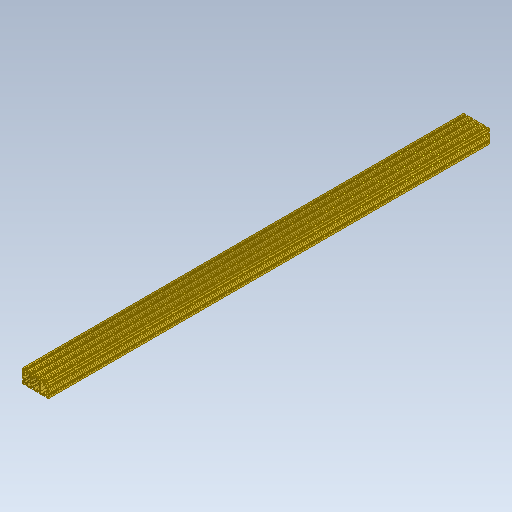
# Autodesk Inventor part: Perfil 60×120 12 rasgos_AST06012012
Saved by Autodesk Inventor 2025.2 (Build 292293000, 293)
## iProperties
Created: 2025-04-07
Part Number: Perfil 60×120 12 rasgos_AST06012012
Material: Ouro
Document SubType Name: Modeling
Designer: Gustavo Sousa
Density: 19.3 g/cm^3
Appearance: Metal quente 2400F
Author: Gustavo Sousa
Autodesk Inventor part; units mm, degrees
ref_plane "YZ Plane" through (0, 0, 0) normal (1, 0, 0) x (0, 1, 0)
ref_plane "XZ Plane" through (0, 0, 0) normal (0, 1, 0) x (-1, 0, 0)
ref_plane "XY Plane" through (0, 0, 0) normal (0, 0, 1) x (1, 0, 0)
sketch "Esboço1" plane through (0, 0, 0) normal (0, 0, 1) x (1, 0, 0)
  line L0 (-60, 30) -> (60, 30) construction
  line L1 (-60, 30) -> (-60, -30) construction
  line L2 (-60, 30) -> (0, 30) construction
  line L3 (-60, 30) -> (-60, 0) construction
  circle A0 centre (-45, 15) radius 5
  line L4 (-45, 15) -> (-60, 30) construction
  line L5 (-60, 30) -> (-30, 30) construction
  line L6 (-52, 22) -> (-38, 22) construction
  line L7 (-49.1, 30) -> (-40.9, 30) construction
  line L8 (-45, 15) -> (-30, 30) construction
  line L9 (-38, 22) -> (-38, 15) construction
  line L10 (-49.1, 30) -> (-49.6, 30) construction
  line L11 (-49.6, 30) -> (-49.6, 29.5)
  line L12 (-49.6, 29.5) -> (-49.1, 29.5)
  line L13 (-49.1, 29.5) -> (-49.1, 30) construction
  line L14 (-49.1, 30) -> (-49.1, 27.8) construction
  line L15 (-49.1, 27.8) -> (-56.2444, 27.8) construction
  arc A1 (-59.5, 30) -> (-60, 29.5) centre (-59.5, 29.5) ccw
  line L16 (-56.2444, 27.8) -> (-50.4444, 22) construction
  arc A2 (-55.0373, 27.8) -> (-55.3908, 26.9464) centre (-55.0373, 27.3) ccw
  arc A3 (-50.5908, 22.1464) -> (-50.2373, 22) centre (-50.2373, 22.5) ccw
  line L17 (-55.0373, 27.8) -> (-49.1, 27.8)
  line L18 (-55.3908, 26.9464) -> (-50.5908, 22.1464)
  line L19 (-50.2373, 22) -> (-45, 22)
  line L20 (-59.5, 30) -> (-49.6, 30)
  line L21 (-39.5556, 22) -> (-33.7556, 27.8) construction
  line L22 (-40.9, 30) -> (-40.4, 30) construction
  line L23 (-40.4, 30) -> (-40.4, 29.5)
  line L24 (-40.4, 29.5) -> (-40.9, 29.5)
  line L25 (-40.9, 29.5) -> (-40.9, 30) construction
  line L26 (-40.9, 30) -> (-40.9, 27.8) construction
  line L27 (-40.9, 27.8) -> (-33.7556, 27.8) construction
  arc A4 (-34.6092, 26.9464) -> (-34.9627, 27.8) centre (-34.9627, 27.3) ccw
  line L28 (-49.1, 29.5) -> (-49.1, 27.8)
  line L29 (-40.9, 29.5) -> (-40.9, 27.8)
  arc A5 (-39.7627, 22) -> (-39.4092, 22.1464) centre (-39.7627, 22.5) ccw
  line L30 (-45, 22) -> (-39.7627, 22)
  line L31 (-39.4092, 22.1464) -> (-34.6092, 26.9464)
  line L32 (-34.9627, 27.8) -> (-40.9, 27.8)
  line L33 (-30, 30) -> (-30, 28.4444) construction
  line L34 (-38, 15) -> (-40, 15) construction
  line L35 (-38, 20.4444) -> (-30, 28.4444) construction
  line L36 (-38, 20.4444) -> (-38, 15) construction
  line L37 (-45, 20) -> (-45, 22)
  line L38 (-40.4, 30) -> (-30, 30)
  arc A6 (-37.8536, 20.5908) -> (-38, 20.2373) centre (-37.5, 20.2373) ccw
  line L39 (-38, 20.2373) -> (-38, 15)
  line L40 (-37.8536, 20.5908) -> (-30, 28.4444)
  arc A7 (-40, 15) -> (-38, 15) centre (-39, 15) ccw
  line L41 (-52, 22) -> (-52, 15) construction
  line L42 (-60, 0) -> (-60, 30) construction
  line L43 (-60, 19.1) -> (-60, 10.9) construction
  line L44 (-45, 15) -> (-60, 0) construction
  line L45 (-52, 15) -> (-52, 8) construction
  line L46 (-60, 19.1) -> (-59.5, 19.1) construction
  line L47 (-59.5, 19.1) -> (-59.5, 19.6)
  line L48 (-59.5, 19.6) -> (-60, 19.6)
  line L49 (-60, 19.6) -> (-60, 19.1) construction
  line L50 (-60, 19.6) -> (-60, 29.5)
  line L51 (-60, 19.1) -> (-57.8, 19.1) construction
  line L52 (-57.8, 19.1) -> (-57.8, 26.2444) construction
  line L53 (-59.5, 19.1) -> (-57.8, 19.1)
  line L54 (-57.8, 26.2444) -> (-52, 20.4444) construction
  line L55 (-52, 20.4444) -> (-52, 15) construction
  line L56 (-52, 8) -> (-45, 8) construction
  line L57 (-45, 15) -> (-45, 10) construction
  line L58 (-45, 10) -> (-45, 8) construction
  arc A8 (-45, 8) -> (-45, 10) centre (-45, 9) ccw
  line L59 (-60, 10.9) -> (-59.5, 10.9) construction
  line L60 (-59.5, 10.9) -> (-59.5, 10.4)
  line L61 (-59.5, 10.4) -> (-60, 10.4)
  line L62 (-60, 10.4) -> (-60, 10.9) construction
  line L63 (-60, 10.4) -> (-60, 0)
  line L64 (-60, 10.9) -> (-57.8, 10.9) construction
  line L65 (-57.8, 10.9) -> (-57.8, 3.7556) construction
  line L66 (-57.8, 3.7556) -> (-52, 9.5556) construction
  line L67 (-52, 15) -> (-52, 9.5556) construction
  line L68 (-60, 0) -> (-58.4444, 0)
  line L69 (-59.5, 10.9) -> (-57.8, 10.9)
  line L70 (-50.4444, 8) -> (-58.4444, 0) construction
  arc A9 (-56.9464, 25.3908) -> (-57.8, 25.0373) centre (-57.3, 25.0373) ccw
  arc A10 (-52, 20.2373) -> (-52.1464, 20.5908) centre (-52.5, 20.2373) ccw
  arc A11 (-52.1464, 9.4092) -> (-52, 9.7627) centre (-52.5, 9.7627) ccw
  arc A12 (-57.8, 4.9627) -> (-56.9464, 4.6092) centre (-57.3, 4.9627) ccw
  arc A13 (-50.2373, 8) -> (-50.5908, 7.8536) centre (-50.2373, 7.5) ccw
  line L71 (-58.4444, 0) -> (-50.5908, 7.8536)
  line L72 (-56.9464, 4.6092) -> (-52.1464, 9.4092)
  line L73 (-50.2373, 8) -> (-45, 8)
  line L74 (-57.8, 10.9) -> (-57.8, 4.9627)
  line L75 (-52, 9.7627) -> (-52, 20.2373)
  line L76 (-52.1464, 20.5908) -> (-56.9464, 25.3908)
  line L77 (-57.8, 25.0373) -> (-57.8, 19.1)
  line L78 (-45, 15) -> (-50, 15) construction
  line L79 (-50, 15) -> (-52, 15)
  line L80 (-30, 30) -> (0, 30) construction
  line L81 (-30, 30) -> (-15, 30) construction
  circle A14 centre (-15, 15) radius 5
  line L82 (-15, 15) -> (-30, 30) construction
  line L83 (-15, 15) -> (0, 30) construction
  line L84 (-22, 22) -> (-8, 22) construction
  line L85 (-19.1, 30) -> (-10.9, 30) construction
  line L86 (-22, 22) -> (-22, 15) construction
  line L87 (-8, 22) -> (-8, 15) construction
  line L88 (-15, 15) -> (-10, 15) construction
  line L89 (-10, 15) -> (-8, 15) construction
  arc A15 (-10, 15) -> (-8, 15) centre (-9, 15) ccw
  line L90 (-22, 15) -> (-22, 8) construction
  line L91 (-15, 15) -> (-15, 10)
  line L92 (-15, 10) -> (-15, 8) construction
  line L93 (-22, 8) -> (-15, 8) construction
  arc A16 (-15, 8) -> (-15, 10) centre (-15, 9) ccw
  line L94 (-22, 0) -> (-22, 8)
  line L95 (-20, 8) -> (-20, 0) construction
  line L96 (-30, 28.4444) -> (-22, 20.4444) construction
  line L97 (-22, 20.4444) -> (-22, 8) construction
  line L98 (-20, 8) -> (-15, 8) construction
  line L99 (-19.1, 30) -> (-19.6, 30) construction
  line L100 (-19.6, 30) -> (-19.6, 29.5)
  line L101 (-19.6, 29.5) -> (-19.1, 29.5)
  line L102 (-19.1, 29.5) -> (-19.1, 30) construction
  line L103 (-30, 30) -> (-19.6, 30)
  line L104 (-19.1, 30) -> (-19.1, 27.8) construction
  line L105 (-19.1, 27.8) -> (-26.2444, 27.8) construction
  line L106 (-19.1, 29.5) -> (-19.1, 27.8)
  line L107 (-26.2444, 27.8) -> (-20.4444, 22) construction
  line L108 (-20.4444, 22) -> (-15, 22) construction
  arc A17 (-25.0373, 27.8) -> (-25.3908, 26.9464) centre (-25.0373, 27.3) ccw
  arc A18 (-20.5908, 22.1464) -> (-20.2373, 22) centre (-20.2373, 22.5) ccw
  line L109 (-19.1, 27.8) -> (-25.0373, 27.8)
  line L110 (-25.3908, 26.9464) -> (-20.5908, 22.1464)
  line L111 (-20.2373, 22) -> (-15, 22)
  arc A19 (-22, 20.2373) -> (-22.1464, 20.5908) centre (-22.5, 20.2373) ccw
  line L112 (-30, 28.4444) -> (-22.1464, 20.5908)
  line L113 (-22, 20.2373) -> (-22, 8)
  line L114 (-10.9, 30) -> (0, 30) construction
  line L115 (-10.9, 30) -> (-10.4, 30) construction
  line L116 (-10.4, 30) -> (-10.4, 29.5)
  line L117 (-10.4, 29.5) -> (-10.9, 29.5)
  line L118 (-10.9, 29.5) -> (-10.9, 30) construction
  line L119 (-10.9, 30) -> (-10.9, 27.8)
  line L120 (-10.9, 27.8) -> (-3.7556, 27.8) construction
  line L121 (-3.7556, 27.8) -> (-9.5556, 22) construction
  arc A20 (-4.6092, 26.9464) -> (-4.9627, 27.8) centre (-4.9627, 27.3) ccw
  arc A21 (-9.7627, 22) -> (-9.4092, 22.1464) centre (-9.7627, 22.5) ccw
  line L122 (-15, 22) -> (-9.7627, 22)
  line L123 (-9.4092, 22.1464) -> (-4.6092, 26.9464)
  line L124 (-4.9627, 27.8) -> (-10.9, 27.8)
  line L125 (-10.4, 30) -> (0, 30)
  line L126 (0, 30) -> (0, 28.4444)
  line L127 (-8, 20.4444) -> (0, 28.4444)
  line L128 (-8, 20.4444) -> (-8, 15)
  arc A22 (-19.5, 8) -> (-20, 7.5) centre (-19.5, 7.5) ccw
  line L129 (-19.5, 8) -> (-15, 8)
  line L130 (-20, 7.5) -> (-20, 0)
  line L131 (-22, 0) -> (-20, 0)
  point P0 (0, 0)
  point P1 (-45, 30)
  point P2 (-45, 30)
  point P3 (-40.9, 28.9)
  point P4 (-60, 15)
  point P5 (-45, 9)
  point P6 (-60, 15)
  point P7 (-15, 30)
  point P8 (-9, 15)
  dimension "d0" = 120
  dimension "d2" = 60
  dimension "d10" = 45
  dimension "d12" = 10
  dimension "d13" = 30
  dimension "d14" = 8
  dimension "d15" = 8.2
  dimension "quadrado" = 0.5
  dimension "espessura" = 2.2
  dimension "arco" = 0.5
  dimension "d20" = 1.1
  dimension "d21" = 1.1
  dimension "d22" = 1.1
  dimension "d26" = 1.1
  dimension "d33" = 10
  dimension "d35" = 2
  dimension "d37" = 2
  constraints: 264 end point, 48 point on circle, 45 point on line, 41 collinear, 39 tangent, 31 equal length, 24 horizontal, 23 centre point, 21 parallel, 21 vertical, 16 equal radius, 15 midpoint, 9 horizontal alignment, 9 perpendicular, 5 coincident, 5 vertical alignment
  measures "d0" distance of L0.start L0.end
  measures "d2" distance of L0.start L1.end
  measures "d10" horizontal distance of point (0, 0) L4.start
  measures "d12" diameter of A0
  measures "d13" distance of L0.start L5.end
  measures "d14" distance between parallel lines of L0 L6
  measures "d15" distance of L7.start L7.end
  measures "quadrado" distance of L12.end L7.start
  measures "espessura" distance between parallel lines of L2 L15
  measures "arco" radius of A1
  measures "d20" distance between parallel lines of L4 L16
  measures "d21" distance between parallel lines of L8 L21
  measures "d22" distance between parallel lines of L8 L35
  measures "d26" distance between parallel lines of L44 L70
  measures "d33" diameter of A14
  measures "d35" distance edge to line of A14 L84
  measures "d37" distance between parallel lines of L94 L95
extrude "Extrusão4" add sketch "Esboço1" along normal mid plane 2000 contours A0 L37 L30 A5 L31 A4 L32 L29 L24 L23 L38 L103 L100 L101 L106 L109 A17 L110 A18 L111 L122 A21 L123 A20 L124 L119 L117 L116 L125 L126 L127 L128 A15 A14 A16 L129 A22 L130 L131 L94 L113 A19 L112 L40 A6 L39 A7 | A0 L79 L75 A10 L76 A9 L77 L53 L47 L48 L50 A1 L20 L11 L12 L28 L17 A2 L18 A3 L19 L37 | A8 L73 A13 L71 L68 L63 L61 L60 L69 L74 A12 L72 A11 L75 L79 A0
mirror "Espelhar5" about plane through (0, 0, 0) normal (0, 1, 0) of "Extrusão4"
mirror "Espelhar6" about plane through (0, 0, 0) normal (1, 0, 0) of "Extrusão4", "Espelhar5"
fillet "Arredondamento1" radius 1 8 edges at (-30, -28.4444, 0) (0, -28.4444, 0) (30, -28.4444, 0) (30, 28.4444, 0) (0, 28.4444, 0) (-30, 28.4444, 0) (-58.4444, 0, 0) (58.4444, 0, 0)
equation "\"d20\" = 0.5 * espessura"
equation "\"d21\" = 0.5 * espessura"
equation "\"d22\" = 0.5 * espessura"
